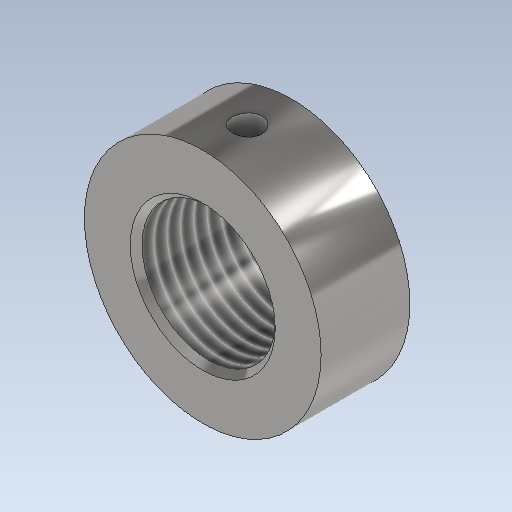
# Autodesk Inventor part: Гайка шток
Saved by Autodesk Inventor 2021 (Build 250183000, 183)
## iProperties
Created: 2020-12-01
Part Number: Гайка шток
Material: Сталь, высокопрочная, низколегированная
Document SubType Name: Modeling
Designer: Тимоха
Mass: 832.316 g
Surface Area: 204.229 cm^2
Volume: 106.027 cm^3
Density: 7.85 g/cm^3
Appearance: Сталь — полированная
Author: Тимоха
Autodesk Inventor part; units mm, degrees
ref_plane "YZ Plane" through (0, 0, 0) normal (1, 0, 0) x (0, 1, 0)
ref_plane "XZ Plane" through (0, 0, 0) normal (0, 1, 0) x (-1, 0, 0)
ref_plane "XY Plane" through (0, 0, 0) normal (0, 0, 1) x (1, 0, 0)
sketch "Эскиз1" plane through (0, 0, 0) normal (0, 0, 1) x (1, 0, 0)
  circle A0 centre (0, 0) radius 40
  circle A1 centre (0, 0) radius 22.5
  dimension "d0" = 80
  dimension "d1" = 45
  constraints: 2 centre point, 2 coincident
  measures "d0" diameter of A0
  measures "d1" diameter of A1
extrude "Выдавливание1" add sketch "Эскиз1" along normal blind 30
sketch "Эскиз2" plane through (0, 0, 0) normal (1, 0, 0) x (0, 1, 0)
  line L0 (40, 0) -> (-40, 0)
  line L1 (22.5, 30) -> (22.5, 0)
  line L2 (22.5, 0) -> (22.5, -6)
  line L3 (22.5, -6) -> (27.5, -6)
  arc A0 (32.491841, 1.501959) -> (29.238817, 0.515685) centre (31.17119, 0) ccw
  line L4 (27.5, -6) -> (29.238817, 0.515685)
  line L5 (34.2, 0) -> (32.491841, 1.501959)
  line L6 (0, -13.2) -> (0, 37.2)
  point P0 (0, 0)
  point P1 (29.101198, 0)
  dimension "d4" = 5
  dimension "d5" = 6
  dimension "d6" = 4
  dimension "d9" = 27.5
  dimension "d10" = 29.23882
  constraints: 9 end point, 2 point on circle, 2 point on line, 2 tangent, 1 centre point, 1 perpendicular, 1 vertical
  measures "d4" distance of L2.end L3.end
  measures "d5" distance of L1.end L2.end
  measures "d6" diameter of A0
  measures "d9" distance from line of L3.end L6
  measures "d10" distance from line of L4.end L6
revolve "Вращение1" add sketch "Эскиз2" angle 360 about axis through (0, 0, -10) along (0, 0, 1) contours L4 L3 L2 L0
revolve "Вращение2" cut sketch "Эскиз2" angle 360 about axis through (0, 0, -10) along (0, 0, 1) contours L0 L4 A0 L5
chamfer "Фаска1" distance 2 angle 45 2 edges at (0, -22.5, -6) (-22.5, 0, 30)
sketch "Эскиз3" plane through (0, 0, 0) normal (1, 0, 0) x (0, 1, 0)
  line L0 (40, 0) -> (40, 30)
  line L1 (40, 15) -> (26.875653, 15)
  line L2 (40, 15) -> (40, 20)
  line L3 (40, 20) -> (30, 20)
  line L4 (30, 20) -> (26.606861, 14.569843)
  point P0 (0, 0)
  dimension "d14" = 10
  dimension "d15" = 58
  constraints: 8 end point, 1 horizontal, 1 midpoint, 1 perpendicular, 1 point on line
  measures "d14" distance of L2.end L3.end
  measures "d15" angle of L1 L4
revolve "Вращение3" cut sketch "Эскиз3" angle 360 about axis through (0, 40, 15) along (0, -1, 0)
thread "Резьба1" size "M45x4.5" class "6H" standard "ANSI Metric M Profile" full length
